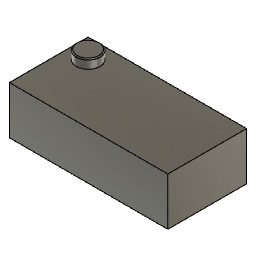
Blocco legov6 (Autodesk Fusion 360 design; units mm, degrees)
Autodesk Fusion 360 part; units mm, degrees
sketch "Sketch1" plane through (0, 0, 0) normal (0, 0, 1) x (1, 0, 0)
  line L0 (0, 0) -> (31.8, 0)
  line L1 (31.8, 0) -> (31.8, 15.8)
  line L2 (31.8, 15.8) -> (0, 15.8)
  line L3 (0, 15.8) -> (0, 0)
  dimension "d3" = 31.8
  dimension "d4" = 15.8
  constraint horizontal L0
  constraint vertical L1
  constraint horizontal L2
  constraint vertical L3
  constraint coincident L0.start L3.end
  measures "d3" distance of L1.end L2.end
  measures "d4" distance of L0.end L1.end
extrude "Extrude1" add sketch "Sketch1" along normal blind 9.6
shell "Shell1" thickness 1.2 removed faces 1 at (21.2, 5.2667, 0)
sketch "Sketch2" plane through (0, 0, 9.6) normal (0, 0, 1) x (-1, 0, 0)
  line L0 (0, -15.8) -> (0, 0)
  line L1 (0, 0) -> (-31.8, 0)
  line L2 (-31.8, 0) -> (-31.8, -15.8)
  line L3 (-31.8, -15.8) -> (0, -15.8)
  circle A0 centre (-3.9, -11.9) radius 2.4
  dimension "d8" = 4.8
  dimension "d9" = 3.9
  dimension "d10" = 3.9
  measures "d8" diameter of A0
  measures "d9" distance of L0 A0.centre
  measures "d10" distance of L3 A0.centre
extrude "Extrude2" add sketch "Sketch2" along normal blind 1.8 contours A0
fillet "Fillet1" radius 0.2 1 edges at (6.1376, 12.7679, 11.4)
equation "d3 = ( 3.9 * 2 ) * 1 mm + ( 8.0 * ( n_orizzontale - 1 ) ) * 1 mm"
equation "d4 = ( 3.9 * 2 ) * 1 mm + ( 8.0 * ( n_verticale - 1 ) ) * 1 mm"
equation "d15 = n_orizzontale"
equation "d16 = n_verticale"
equation "n_orizzontale = 4"
equation "n_verticale = 2"
